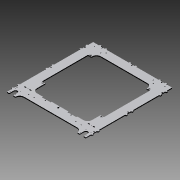
# Autodesk Inventor part: BACK PLATE
Saved by Autodesk Inventor 2013 (Build 170138000, 138)
## iProperties
Created: 2014-06-19
Part Number: BACK PLATE
Material: Generic
Document SubType Name: Modeling
Designer: employee
Density: 1 g/cm^3
Author: employee
Autodesk Inventor part; units mm, degrees
ref_plane "YZ Plane" through (0, 0, 0) normal (1, 0, 0) x (0, 1, 0)
ref_plane "XZ Plane" through (0, 0, 0) normal (0, 1, 0) x (-1, 0, 0)
ref_plane "XY Plane" through (0, 0, 0) normal (0, 0, 1) x (1, 0, 0)
sketch "Sketch1" plane through (0, 0, 0) normal (0, 0, 1) x (1, 0, 0)
  line L0 (-161.5, 187.5) -> (161.5, 187.5)
  line L1 (161.5, 187.5) -> (161.5, -187.5)
  line L2 (161.5, -187.5) -> (-161.5, -187.5)
  line L3 (-161.5, -187.5) -> (-161.5, 187.5)
  line L4 (-231.5, 237.5) -> (231.5, 237.5)
  line L5 (231.5, 237.5) -> (231.5, -268.215)
  line L6 (-231.5, -268.215) -> (-231.5, 237.5)
  line L7 (-181.5, -268.215) -> (-181.5, -243.215)
  line L8 (-181.5, -243.215) -> (181.5, -243.215)
  line L9 (181.5, -243.215) -> (181.5, -268.215)
  line L10 (231.5, -268.215) -> (181.5, -268.215)
  line L11 (-181.5, -268.215) -> (-231.5, -268.215)
  point P0 (0, 0)
  point P1 (-161.5, 0)
  point P2 (0, -187.5)
  dimension "d0" = 323
  dimension "d2" = 375
  dimension "d4" = 70
  dimension "d5" = 50
  dimension "d6" = 70
  dimension "d7" = 55.715
  dimension "d8" = 25
  dimension "d9" = 50
  dimension "d10" = 50
  constraints: 24 end point, 6 parallel, 5 perpendicular, 2 horizontal, 2 horizontal alignment, 2 midpoint, 1 vertical alignment
  measures "d0" distance of L1.end L2.end
  measures "d2" distance of L2.end L0.start
  measures "d4" distance between parallel lines of L3 L6
  measures "d5" distance between parallel lines of L4 L0
  measures "d6" distance between parallel lines of L5 L1
  measures "d7" distance between parallel lines of L2 L8
  measures "d8" distance between parallel lines of L8 L11
  measures "d9" distance of L7.start L6.start
  measures "d10" distance of L5.end L9.end
extrude "Extrusion1" add sketch "Sketch1" along normal blind 5.715
sketch "Sketch2" plane through (0, 0, 5.715) normal (0, 0, 1) x (1, 0, 0)
  line L0 (161.5, -187.5) -> (-161.5, -187.5) projected
  line L1 (-161.5, -187.5) -> (-161.5, 187.5) projected
  line L2 (-231.5, 237.5) -> (-231.5, -268.215) projected
  line L3 (231.5, -268.215) -> (231.5, 237.5) projected
  line L4 (-161.5, -112.5) -> (-169.5, -112.5)
  line L5 (-169.5, -112.5) -> (-169.5, -122.5)
  line L6 (-169.5, -122.5) -> (-173.5, -122.5)
  line L7 (-173.5, -122.5) -> (-173.5, -112.5)
  line L8 (-173.5, -112.5) -> (-181.5, -112.5)
  line L9 (-181.5, -112.5) -> (-181.5, 157.5)
  line L10 (-181.5, 157.5) -> (-173.5, 157.5)
  line L11 (-173.5, 157.5) -> (-173.5, 167.5)
  line L12 (-173.5, 167.5) -> (-169.5, 167.5)
  line L13 (-169.5, 167.5) -> (-169.5, 157.5)
  line L14 (-169.5, 157.5) -> (-161.5, 157.5)
  point P0 (0, 0)
  dimension "d13" = 290
  dimension "d15" = 10
  dimension "d16" = 20
  dimension "d17" = 75
  dimension "d18" = 4
  constraints: 22 end point, 6 equal length, 5 parallel, 5 perpendicular, 2 point on line, 1 collinear
  measures "d13" distance between parallel lines of L12 L6
  measures "d15" distance of L10.end L11.end
  measures "d16" distance between parallel lines of L1 L9
  measures "d17" distance between parallel lines of L0 L4
  measures "d18" distance between parallel lines of L7 L5
extrude "Extrusion2" cut sketch "Sketch2" against normal through all
sketch "Sketch3" plane through (0, 0, 5.715) normal (0, 0, 1) x (1, 0, 0)
  line L0 (-169.5, -112.5) -> (-169.5, -122.5) projected
  line L1 (-169.5, -122.5) -> (-173.5, -122.5) projected
  line L2 (-173.5, -122.5) -> (-173.5, -112.5) projected
  line L3 (-173.5, 157.5) -> (-173.5, 167.5) projected
  line L4 (-173.5, 167.5) -> (-169.5, 167.5) projected
  line L5 (-169.5, 167.5) -> (-169.5, 157.5) projected
  line L6 (-175.5, 164.5) -> (-177, 164.5)
  line L7 (-177, 164.5) -> (-177, 160.5)
  line L8 (-177, 160.5) -> (-175.5, 160.5)
  line L9 (-175.5, 160.5) -> (-175.5, 164.5)
  line L10 (-167.5, 164.5) -> (-166, 164.5)
  line L11 (-166, 164.5) -> (-166, 160.5)
  line L12 (-166, 160.5) -> (-167.5, 160.5)
  line L13 (-167.5, 160.5) -> (-167.5, 164.5)
  line L14 (-175.5, -115.5) -> (-177, -115.5)
  line L15 (-177, -115.5) -> (-177, -119.5)
  line L16 (-177, -119.5) -> (-175.5, -119.5)
  line L17 (-175.5, -119.5) -> (-175.5, -115.5)
  line L18 (-167.5, -115.5) -> (-166, -115.5)
  line L19 (-166, -115.5) -> (-166, -119.5)
  line L20 (-166, -119.5) -> (-167.5, -119.5)
  line L21 (-167.5, -119.5) -> (-167.5, -115.5)
  line L22 (-175.5, -117.5) -> (-167.5, -117.5)
  line L23 (-175.5, 162.5) -> (-167.5, 162.5)
  point P0 (0, 0)
  point P1 (-173.5, 162.5)
  point P2 (-169.5, 162.5)
  point P3 (-173.5, -117.5)
  point P4 (-169.5, -117.5)
  point P5 (-171.5, -117.5)
  point P6 (-171.5, -122.5)
  point P7 (-171.5, 162.5)
  point P8 (-171.5, 167.5)
  dimension "d22" = 8
  dimension "d24" = 1.5
  dimension "d25" = 4
  constraints: 36 end point, 12 midpoint, 9 parallel, 7 equal length, 5 perpendicular, 4 horizontal, 4 horizontal alignment, 2 vertical alignment
  measures "d22" distance of L23.start L23.end
  measures "d24" distance of L15.end L16.end
  measures "d25" distance of L14.end L15.end
extrude "Extrusion3" cut sketch "Sketch3" against normal through all contours L9 L8 L7 L6 | L10 L11 L12 L13 | L17 L16 L15 L14 | L18 L19 L20 L21
mirror "Mirror1" about plane through (0, 0, 0) normal (1, 0, 0) of "Extrusion2", "Extrusion3"
fillet "Fillet1" radius 25 6 edges at (-161.5, 187.5, 2.8575) (161.5, 187.5, 2.8575) (161.5, -187.5, 2.8575) (-161.5, -187.5, 2.8575) (-181.5, -243.215, 2.8575) (181.5, -243.215, 2.8575)
fillet "Fillet3" radius 2 12 edges at (-181.5, -112.5, 2.8575) (-161.5, -112.5, 2.8575) (181.5, -112.5, 2.8575) (161.5, -112.5, 2.8575) (181.5, 157.5, 2.8575) (161.5, 157.5, 2.8575) (-161.5, 157.5, 2.8575) (-181.5, 157.5, 2.8575) (-181.5, -268.2149, 2.8575) (-181.5, -268.215, 2.8575) (181.5, -268.2149, 2.8575) (181.5, -268.215, 2.8575)
sketch "Sketch5" plane through (0, 0, 5.715) normal (0, 0, 1) x (1, 0, 0)
  line L0 (231.5, 237.5) -> (-231.5, 237.5) projected
  line L1 (-1.5, 237.5) -> (1.5, 237.5)
  line L2 (1.5, 237.5) -> (1.5, 229.215)
  line L3 (1.5, 229.215) -> (-1.5, 229.215)
  line L4 (-1.5, 229.215) -> (-1.5, 237.5)
  line L5 (-2.75, 233.215) -> (2.75, 233.215)
  line L6 (2.75, 233.215) -> (2.75, 231.215)
  line L7 (2.75, 231.215) -> (-2.75, 231.215)
  line L8 (-2.75, 231.215) -> (-2.75, 233.215)
  point P0 (0, 0)
  point P1 (0, 237.5)
  point P2 (0, 233.215)
  point P3 (0, 237.5)
  dimension "d30" = 2
  dimension "d32" = 5.5
  dimension "d33" = 3
  dimension "d34" = 8.285
  dimension "d35" = 6.285
  constraints: 16 end point, 4 midpoint, 4 parallel, 2 horizontal, 2 perpendicular, 1 point on line, 1 vertical alignment
  measures "d30" distance of L5.end L6.end
  measures "d32" distance of L6.end L7.end
  measures "d33" distance of L2.end L3.end
  measures "d34" distance between parallel lines of L0 L3
  measures "d35" distance between parallel lines of L7 L0
extrude "Extrusion4" cut sketch "Sketch5" against normal blind 5.715
sketch "Sketch6" plane through (0, 0, 5.715) normal (0, 0, 1) x (1, 0, 0)
  line L0 (1.5, 229.215) -> (-1.5, 229.215) projected
  line L1 (-1.5, 237.5) -> (-231.5, 237.5) projected
  line L2 (231.5, 237.5) -> (1.5, 237.5) projected
  line L3 (-12.5, 237.5) -> (-22.5, 237.5)
  line L4 (-22.5, 237.5) -> (-22.5, 243.215)
  line L5 (-22.5, 243.215) -> (-12.5, 243.215)
  line L6 (-12.5, 243.215) -> (-12.5, 237.5)
  line L7 (12.5, 237.5) -> (22.5, 237.5)
  line L8 (22.5, 237.5) -> (22.5, 243.215)
  line L9 (22.5, 243.215) -> (12.5, 243.215)
  line L10 (12.5, 243.215) -> (12.5, 237.5)
  line L11 (-12.5, 243.215) -> (12.5, 243.215)
  point P0 (0, 0)
  point P1 (0, 243.215)
  point P2 (0, 229.215)
  dimension "d38" = 5.715
  dimension "d40" = 10
  dimension "d41" = 25
  constraints: 18 end point, 4 parallel, 2 collinear, 2 horizontal, 2 midpoint, 2 perpendicular, 2 point on line, 1 vertical alignment
  measures "d38" distance of L9.end L7.start
  measures "d40" distance of L8.end L9.end
  measures "d41" distance of L5.end L9.end
extrude "Extrusion5" add sketch "Sketch6" against normal up to surface (5.715 mm away)
pattern_linear "Rectangular Pattern1" count 3 spacing 175 along (-1, 0, 0) of "Extrusion4", "Extrusion5" first direction both ways yes
sketch "Sketch7" plane through (0, 0, 5.715) normal (0, 0, 1) x (1, 0, 0)
  line L0 (-231.5, 237.5) -> (-231.5, -268.215) projected
  line L1 (1.5, 229.215) -> (-1.5, 229.215) projected
  line L2 (-1.5, 229.215) -> (-1.5, 231.215) projected
  line L3 (-1.5, 231.215) -> (-2.75, 231.215) projected
  line L4 (-2.75, 231.215) -> (-2.75, 233.215) projected
  line L5 (-1.5, 233.215) -> (-1.5, 237.5) projected
  line L6 (-223.215, -13.8575) -> (-223.215, -16.8575)
  line L7 (-231.5, -16.8575) -> (-231.5, -13.8575)
  line L8 (-227.215, -12.6075) -> (-225.215, -12.6075)
  line L9 (-225.215, -18.1075) -> (-227.215, -18.1075)
  line L10 (-223.215, -16.8575) -> (-225.215, -16.8575)
  line L11 (-227.215, -16.8575) -> (-231.5, -16.8575)
  line L12 (-227.215, -18.1075) -> (-227.215, -16.8575)
  line L13 (-227.215, -13.8575) -> (-227.215, -12.6075)
  line L14 (-231.5, -13.8575) -> (-227.215, -13.8575)
  line L15 (-225.215, -13.8575) -> (-223.215, -13.8575)
  line L16 (-225.215, -12.6075) -> (-225.215, -13.8575)
  line L17 (-225.215, -16.8575) -> (-225.215, -18.1075)
  point P0 (0, 0)
  point P1 (-231.5, -15.3575)
  constraints: 24 end point, 10 parallel, 6 equal length, 4 perpendicular, 3 horizontal, 2 horizontal alignment, 2 midpoint, 2 vertical alignment, 1 point on line
extrude "Extrusion6" cut sketch "Sketch7" against normal through all
sketch "Sketch8" plane through (0, 0, 5.715) normal (0, 0, 1) x (1, 0, 0)
  line L0 (-223.215, -13.8575) -> (-223.215, -16.8575) projected
  line L1 (-231.5, -16.8575) -> (-231.5, -268.215) projected
  line L2 (-12.5, 243.215) -> (-22.5, 243.215) projected
  line L3 (-22.5, 243.215) -> (-22.5, 237.5) projected
  line L4 (-231.5, 237.5) -> (-231.5, -13.8575) projected
  line L5 (-231.5, -2.8575) -> (-237.215, -2.8575)
  line L6 (-237.215, -2.8575) -> (-237.215, 7.1425)
  line L7 (-237.215, 7.1425) -> (-231.5, 7.1425)
  line L8 (-231.5, 7.1425) -> (-231.5, -2.8575)
  line L9 (-231.5, -27.8575) -> (-237.215, -27.8575)
  line L10 (-237.215, -27.8575) -> (-237.215, -37.8575)
  line L11 (-237.215, -37.8575) -> (-231.5, -37.8575)
  line L12 (-231.5, -37.8575) -> (-231.5, -27.8575)
  line L13 (-237.215, -2.8575) -> (-237.215, -27.8575)
  line L14 (-12.5, 243.215) -> (12.5, 243.215)
  point P0 (0, 0)
  point P1 (-237.215, -15.3575)
  point P2 (-223.215, -15.3575)
  constraints: 20 end point, 5 parallel, 4 equal length, 3 perpendicular, 2 horizontal, 2 midpoint, 2 point on line, 1 horizontal alignment
extrude "Extrusion7" add sketch "Sketch8" against normal up to surface (5.715 mm away)
pattern_linear "Rectangular Pattern2" count 3 spacing 200 along (0, -1, 0) of "Extrusion6", "Extrusion7" first direction both ways yes
mirror "Mirror2" about plane through (0, 0, 0) normal (1, 0, 0) of "Extrusion6", "Extrusion7", "Rectangular Pattern2"
sketch "Sketch9" plane through (0, 0, 0) normal (0, 0, -1) x (-1, 0, 0)
  line L0 (-231.5, -237.8575) -> (-231.5, -268.215) projected
  line L1 (-231.5, -268.215) -> (-183.4258, -268.215) projected
  line L2 (-222, -258.715) -> (-222, -227.715) construction
  line L3 (-222, -227.715) -> (-191, -227.715) construction
  line L4 (-191, -227.715) -> (-191, -258.715) construction
  line L5 (-191, -258.715) -> (-222, -258.715) construction
  circle A0 centre (-222, -227.715) radius 1.5
  arc A1 (-195, -243.215) -> (-218, -243.215) centre (-206.5, -243.215) ccw
  circle A2 centre (-222, -258.715) radius 1.5
  circle A3 centre (-191, -258.715) radius 1.5
  circle A4 centre (-191, -227.715) radius 1.5
  line L6 (-218, -243.215) -> (-218, -268.215)
  line L7 (-195, -243.215) -> (-195, -268.215)
  point P0 (0, 0)
  dimension "d54" = 25
  dimension "d55" = 25
  dimension "d56" = 31
  dimension "d57" = 3
  dimension "d58" = 23
  constraints: 12 end point, 5 centre point, 5 coincident, 3 equal radius, 2 perpendicular, 2 point on circle, 2 point on line, 2 tangent, 1 horizontal, 9 other
  measures "d54" distance from line of point (-206.5, -243.215) L1
  measures "d55" distance from line of point (-206.5, -243.215) L0
  measures "d56" distance of L2.end L3.end
  measures "d57" diameter of A0
  measures "d58" diameter of A1
extrude "Extrusion8" cut sketch "Sketch9" against normal through all
mirror "Mirror3" about plane through (0, 0, 0) normal (1, 0, 0) of "Extrusion8"
sketch "Sketch10" plane through (0, 0, 0) normal (0, 0, -1) x (-1, 0, 0)
  line L0 (-166.5, -193.215) -> (-176.5, -193.215) projected
  line L1 (-166.5, -187.5) -> (-166.5, -193.215) projected
  line L2 (-176.5, -187.5) -> (-166.5, -187.5) projected
  line L3 (-176.5, -187.5) -> (-176.5, -193.215) projected
  line L4 (-196.5, -193.215) -> (-206.5, -193.215) projected
  line L5 (-196.5, -187.5) -> (-196.5, -193.215) projected
  line L6 (-206.5, -187.5) -> (-196.5, -187.5) projected
  line L7 (-206.5, -187.5) -> (-206.5, -193.215) projected
  line L8 (-50, -193.215) -> (-100, -193.215) projected
  line L9 (-50, -187.5) -> (-50, -193.215) projected
  line L10 (-100, -187.5) -> (-50, -187.5) projected
  line L11 (-100, -187.5) -> (-100, -193.215) projected
  line L12 (50, -193.215) -> (100, -193.215) projected
  line L13 (100, -187.5) -> (100, -193.215) projected
  line L14 (100, -187.5) -> (50, -187.5) projected
  line L15 (50, -187.5) -> (50, -193.215) projected
  line L16 (166.5, -193.215) -> (176.5, -193.215) projected
  line L17 (176.5, -187.5) -> (176.5, -193.215) projected
  line L18 (176.5, -187.5) -> (166.5, -187.5) projected
  line L19 (166.5, -187.5) -> (166.5, -193.215) projected
  line L20 (196.5, -193.215) -> (206.5, -193.215) projected
  line L21 (206.5, -187.5) -> (206.5, -193.215) projected
  line L22 (206.5, -187.5) -> (196.5, -187.5) projected
  line L23 (196.5, -187.5) -> (196.5, -193.215) projected
  line L24 (-196.5, -190.3575) -> (-176.5, -190.3575)
  line L25 (-50, -190.3575) -> (50, -190.3575)
  line L26 (176.5, -190.3575) -> (196.5, -190.3575)
  circle A0 centre (186.5, -190.3575) radius 1.5
  circle A1 centre (0, -190.3575) radius 1.5
  circle A2 centre (-186.5, -190.3575) radius 1.5
  point P0 (0, 0)
  dimension "d61" = 3
  constraints: 9 midpoint, 6 end point, 3 centre point, 2 equal radius
  measures "d61" diameter of A0
extrude "Extrusion9" cut sketch "Sketch10" against normal through all
sketch "Sketch11" plane through (0, 0, 0) normal (0, 0, -1) x (-1, 0, 0)
  line L0 (50, -187.5) -> (-50, -187.5) projected
  line L1 (-50, -193.215) -> (-100, -193.215) projected
  line L2 (-76.5, -193.215) -> (-73.5, -193.215)
  line L3 (-73.5, -193.215) -> (-73.5, -201.5)
  line L4 (-73.5, -201.5) -> (-76.5, -201.5)
  line L5 (-76.5, -201.5) -> (-76.5, -193.215)
  line L6 (-77.75, -197.5) -> (-72.25, -197.5)
  line L7 (-72.25, -197.5) -> (-72.25, -199.5)
  line L8 (-72.25, -199.5) -> (-77.75, -199.5)
  line L9 (-77.75, -199.5) -> (-77.75, -197.5)
  point P0 (0, 0)
  point P1 (-75, -193.215)
  point P2 (-75, -193.215)
  point P3 (-75, -199.5)
  point P4 (-75, -201.5)
  dimension "d65" = 12
  dimension "d66" = 14
  dimension "d67" = 3
  dimension "d68" = 2
  dimension "d69" = 5.5
  constraints: 16 end point, 4 midpoint, 4 parallel, 2 horizontal, 2 perpendicular, 1 coincident, 1 point on line, 1 vertical alignment
  measures "d65" distance between parallel lines of L0 L8
  measures "d66" distance between parallel lines of L0 L4
  measures "d67" distance of L3.end L4.end
  measures "d68" distance of L6.end L7.end
  measures "d69" distance of L7.end L8.end
extrude "Extrusion10" cut sketch "Sketch11" against normal through all
mirror "Mirror4" about plane through (0, 0, 0) normal (1, 0, 0) of "Extrusion10"
fillet "Fillet4" radius 2 4 edges at (-218, -268.215, 2.8575) (-195, -268.215, 2.8575) (195, -268.215, 2.8575) (218, -268.215, 2.8575)
sketch "Sketch12" plane through (0, 0, 5.715) normal (0, 0, 1) x (1, 0, 0)
  line L0 (-136.5, 187.5) -> (136.5, 187.5) projected
  line L1 (-231.5, 237.5) -> (-231.5, 207.1425) projected
  line L2 (-156.5, -243.215) -> (156.5, -243.215) projected
  line L3 (218, -243.215) -> (218, -266.215) projected
  line L4 (-138, 298.6) -> (-138, -320.8113) construction
  line L5 (-122, -320.8113) -> (-122, 328.2604) construction
  line L6 (-154, 328.2604) -> (-154, -454.7328) construction
  line L7 (-154, -218.215) -> (-122, -218.215) construction
  circle A0 centre (-138, 220.5) radius 2.5
  circle A1 centre (-154, 204.5) radius 2.5
  circle A2 centre (-206.5, 220.5) radius 2.5
  circle A3 centre (-154, -218.215) radius 2.5
  circle A4 centre (-122, -218.215) radius 2.5
  point P0 (0, 0)
  dimension "d73" = 138
  dimension "d74" = 16
  dimension "d75" = 16
  dimension "d76" = 25
  dimension "d77" = 17
  dimension "d78" = 16
  dimension "d79" = 25
  dimension "d80" = 5
  constraints: 8 end point, 5 centre point, 4 equal radius, 4 point on line, 3 parallel, 2 coincident, 1 horizontal alignment, 1 perpendicular
  measures "d73" distance from line of L4 point (0, 0)
  measures "d74" distance between parallel lines of L5 L4
  measures "d75" distance between parallel lines of L6 L4
  measures "d76" distance between parallel lines of L7 L2
  measures "d77" distance from line of A1.centre L0
  measures "d78" horizontal distance of A0.centre A1.centre
  measures "d79" distance from line of L1 A2.centre
  measures "d80" diameter of A2
extrude "Extrusion11" cut sketch "Sketch12" against normal through all
mirror "Mirror5" about plane through (0, 0, 0) normal (1, 0, 0) of "Extrusion11"
sketch "Sketch13" plane through (0, 0, 0) normal (0, 0, -1) x (-1, 0, 0)
  circle A0 centre (0, -190.3575) radius 1.5 projected
  circle A1 centre (0, -198.3575) radius 5
  point P0 (0, 0)
  dimension "d83" = 8
  dimension "d84" = 10
  constraints: 1 centre point, 1 vertical alignment
  measures "d83" distance of A0.centre A1.centre
  measures "d84" diameter of A1
extrude "Extrusion12" cut sketch "Sketch13" against normal through all contours A1
body "Solid1"
